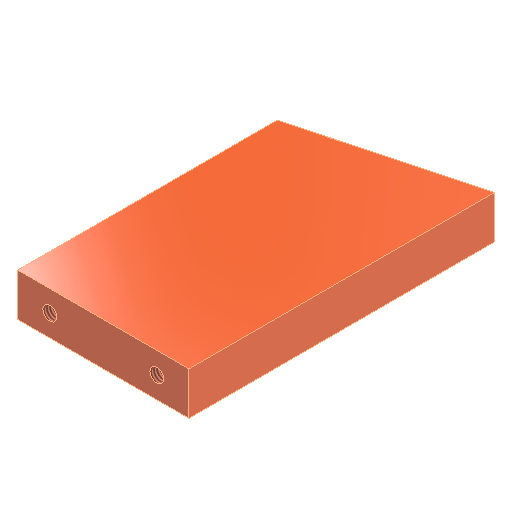
# Autodesk Inventor part: GRJ-03-115
Saved by Autodesk Inventor 2026.1 (Build 301233000, 233)
## iProperties
Company: Gree
Created: 2024-12-19
Part Number: GRJ-03-115
Material: Fenolite OR
Document SubType Name: Modeling
Designer: Willian Pinheiro
Density: 1.38 g/cm^3
Appearance: Suave - Laranja claro
Description: Coluna Montagem
Mass: 35.7397 g
Surface Area: 78.6536 cm^2
Volume: 25.8983 cm^3
Project: GRJ-03
Checked By: Antonio Lucas
Engr Approved By: Antonio Lucas
Mfg Approved By: Anderson Oliveira
Dimensões: 10 x 40 x 72 mm
Total: 1
Author: Willian Pinheiro
Revision Number: 00
Title: Soldagem
Autodesk Inventor part; units mm, degrees
ref_plane "YZ Plane" through (0, 0, 0) normal (1, 0, 0) x (0, 1, 0)
ref_plane "XZ Plane" through (0, 0, 0) normal (0, 1, 0) x (-1, 0, 0)
ref_plane "XY Plane" through (0, 0, 0) normal (0, 0, 1) x (1, 0, 0)
sketch "Esboço1" plane through (0, 0, 0) normal (0, 0, 1) x (1, 0, 0)
  line L0 (-20, -35.65) -> (20, -35.65)
  line L1 (20, -35.65) -> (20, 35.65)
  line L2 (20, 35.65) -> (-20, 35.65)
  line L3 (-20, 35.65) -> (-20, -35.65)
  line L4 (-20, 35.65) -> (20, 35.65)
  circle A0 centre (0, 25.65) radius 5 construction
  circle A1 centre (0, 25.65) radius 28 construction
  circle A2 centre (0, 25.65) radius 74 construction
  line L5 (-20, 6.0541) -> (20, 6.0541) construction
  line L6 (-20, -48.35) -> (20, -48.35) construction
  line L7 (-103.6, 0) -> (103.6, 0) construction
  line L8 (0, -77.95) -> (0, 129.25) construction
  line L9 (-20, 24.932) -> (20, 35.65)
  point P0 (0, 0)
  dimension "d0" = 71.3
  dimension "d1" = 40
  dimension "d41" = 10
  dimension "d42" = 61.3
  dimension "d43" = 56
  dimension "d45" = 84
  dimension "d49" = 15
  dimension "d58" = 10
  constraints: 16 end point, 5 point on line, 3 centre point, 3 parallel, 2 coincident, 2 horizontal, 2 point on circle, 1 midpoint, 1 perpendicular, 1 tangent, 2 other
  measures "d0" distance between parallel lines of L0 L2
  measures "d1" distance of L2.end L1.end
  measures "d41" diameter of A0
  measures "d42" distance from line of L0 A0.centre
  measures "d43" diameter of A1
  measures "d49" angle of L9 L2
  measures "d58" distance from line of A0.centre L4
extrude "Extrusão1" add sketch "Esboço1" along normal mid plane 10
extrude "Extrusão4" cut sketch "Esboço1" along normal through all both and the other way through all contours L3 L2 L9
sketch "Esboço2" plane through (-20, -35.65, -5) normal (0, -1, 0) x (1, 0, 0)
  line L0 (40, 10) -> (40, 0)
  line L1 (40, 5) -> (0, 5) construction
  line L2 (0, 0) -> (0, 10)
  line L3 (0, 0) -> (0, 10) projected
  line L4 (40, 0) -> (40, 10) projected
  line L5 (0, 10) -> (40, 10) construction
  line L6 (20, 10) -> (20, 0) construction
  line L7 (40, 0) -> (0, 0) construction
  point P0 (20, 5)
  point P1 (7.5, 5)
  point P2 (32.5, 5)
  dimension "d9" = 7.5
  dimension "d10" = 7.5
  dimension "d37" = 25
  constraints: 8 end point, 4 midpoint, 2 point on line, 1 symmetric about line
  measures "d9" distance from line of L2 point (7.5, 5)
  measures "d10" distance from line of L0 point (32.5, 5)
  measures "d37" distance of point (32.5, 5) point (7.5, 5)
hole "Furo1" at (-12.5, -35.65, 0) at (12.5, -35.65, 0) direction (0, 1, 0) diameter 3.242 depth 15 tip angle 118 thread size "M4x0.7" class "6H" standard "ISO Metric profile"
sketch "Esboço3" plane through (0, 0, 5) normal (0, 0, 1) x (1, 0, 0)
  point P0 (0, 0)
  point P1 (0, 37.5)
  point P2 (0, 25.65)
hole "Furo2" [suppressed]
sketch "Esboço6" plane through (20, 35.65, 5) normal (-0.258819, 0.9659258, 0) x (0.9659258, 0.258819, 0)
  line L0 (0, 0) -> (0, 10) construction
  line L1 (0, 5) -> (-41.411, 5) construction
  line L2 (-41.411, 0) -> (-41.411, 10) construction
  line L3 (-20.7055, 5) -> (-20.7055, 0) construction
  point P0 (-28.5454, 5)
  point P1 (-30.7055, 5)
  point P2 (-10.7055, 5)
  dimension "d50" = 20
  constraints: 4 end point, 3 midpoint, 2 point on line, 1 symmetric about line, 1 vertical
  measures "d50" distance of point (-10.706, 5) point (-30.706, 5)
hole "Furo3" at (-9.6593, 27.7028, 0) direction (0.258819, -0.9659258, 0) diameter 3.242 depth 15 tip angle 118 countersink diameter 10 countersink angle 90 thread size "M4x0.7" class "6H" standard "ISO Metric profile"
